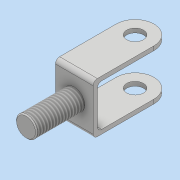
# Autodesk Inventor part: Giá đỡ ròng rọc
Saved by Autodesk Inventor 2018 (Build 220112000, 112)
## iProperties
Created: 2020-08-11
Part Number: Giá đỡ ròng rọc
Material: Generic
Document SubType Name: Modeling
Designer: ASUS
Density: 1 g/cm^3
Appearance: Default
Author: ASUS
Autodesk Inventor part; units mm, degrees
ref_plane "YZ Plane" through (0, 0, 0) normal (1, 0, 0) x (0, 1, 0)
ref_plane "XZ Plane" through (0, 0, 0) normal (0, 1, 0) x (-1, 0, 0)
ref_plane "XY Plane" through (0, 0, 0) normal (0, 0, 1) x (1, 0, 0)
sketch "Sketch1" plane through (0, 0, 0) normal (0, 1, 0) x (-1, 0, 0)
  line L0 (9, 12) -> (-9, 12)
  line L1 (-9, 12) -> (-9, -12)
  line L2 (-9, -12) -> (9, -12)
  line L3 (9, -12) -> (9, 12)
  line L4 (9, 12) -> (-9, -12) construction
  line L5 (-9, 12) -> (9, -12) construction
  point P0 (0, 0)
  dimension "d0" = 24
  dimension "d1" = 18
  constraints: 12 end point, 2 midpoint, 2 parallel, 1 horizontal, 1 perpendicular
  measures "d0" distance of L1.end L0.end
  measures "d1" distance of L1.end L2.end
extrude "Extrusion1" add sketch "Sketch1" along normal blind 2
sketch "Sketch2" plane through (0, 2, 0) normal (0, 1, 0) x (1, 0, 0)
  line L0 (-9, 12) -> (-9, -12) projected
  line L1 (9, -12) -> (9, 12) projected
  line L2 (-9, -12) -> (9, -12)
  line L3 (9, -12) -> (9, -10)
  line L4 (9, -10) -> (-9, -10)
  line L5 (-9, -10) -> (-9, -12)
  line L6 (9, 12) -> (-9, 12) projected
  line L7 (-9, 12) -> (9, 12)
  line L8 (9, 12) -> (9, 10)
  line L9 (9, 10) -> (-9, 10)
  line L10 (-9, 10) -> (-9, 12)
  point P0 (0, 0)
  dimension "d4" = 2
  dimension "d5" = 2
  constraints: 16 end point, 4 parallel, 2 horizontal, 2 perpendicular, 2 point on line
  measures "d4" distance of L3.end L2.end
  measures "d5" distance of L7.end L8.end
extrude "Extrusion2" add sketch "Sketch2" along normal blind 36 contours L6 L1 L9 L0 | L4 L1 L2 L0
sketch "Sketch5" plane through (-9, 0, 12) normal (0, 0, 1) x (1, 0, 0)
  line L0 (0, 29) -> (18, 29)
  line L1 (0, 38) -> (18, 38) projected
  arc A0 (18, 29) -> (0, 29) centre (9, 29) ccw
  circle A1 centre (9, 29) radius 4
  line L2 (0, 0) -> (0, 38) projected
  line L3 (0, 29) -> (0, 38)
  line L4 (18, 38) -> (0, 38) projected
  line L5 (0, 38) -> (18, 38)
  line L6 (18, 38) -> (18, 29)
  point P0 (9, 0)
  dimension "d16" = 9
  dimension "d17" = 8
  constraints: 8 end point, 2 centre point, 2 point on circle, 1 coincident, 1 collinear, 1 horizontal, 1 perpendicular, 1 vertical
  measures "d16" distance between parallel lines of L1 L0
  measures "d17" diameter of A1
extrude "Extrusion4" cut sketch "Sketch5" against normal blind 40 contours A1 L0 | L0 A1 | A0 L1 L6 | A0 L2 L1
sketch "Sketch6" plane through (0, 0, 0) normal (0, -1, 0) x (1, 0, 0)
  circle A0 centre (0, 0) radius 4
  dimension "d20" = 8
  constraints: 1 centre point, 1 coincident
  measures "d20" diameter of A0
extrude "Extrusion5" cut sketch "Sketch6" against normal blind 40
fillet "Fillet1" radius 2 4 edges at (0, 0, 12) (0, 0, -12) (0, 2, 10) (0, 2, -10)
sketch "Sketch11" plane through (0, 2, 0) normal (0, 1, 0) x (1, 0, 0)
  circle A0 centre (0, 0) radius 5
  dimension "d29" = 10
  constraints: 1 centre point, 1 coincident
  measures "d29" diameter of A0
extrude "Extrusion7" add sketch "Sketch11" against normal blind 25
thread "Thread2" size "M10x1.5" class "6g" standard "ANSI Metric M Profile" full length
chamfer "Chamfer1" distance 0.5 angle 45 1 edges at (-5, -23, 0)
body "Solid1"
